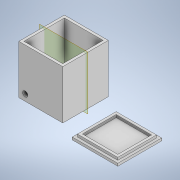
# Autodesk Inventor part: waterBallonHolder
Saved by Autodesk Inventor 2020 (Build 240168000, 168)
## iProperties
Created: 2022-09-13
Part Number: waterBallonHolder
Material: Generic
Document SubType Name: Modeling
Designer: iss
Density: 1 g/cm^3
Appearance: Default
Author: iss
Autodesk Inventor part; units mm, degrees
ref_plane "YZ Plane" through (0, 0, 0) normal (1, 0, 0) x (0, 1, 0)
ref_plane "XZ Plane" through (0, 0, 0) normal (0, 1, 0) x (-1, 0, 0)
ref_plane "XY Plane" through (0, 0, 0) normal (0, 0, 1) x (1, 0, 0)
sketch "Sketch1" plane through (0, 0, 0) normal (0, 1, 0) x (-1, 0, 0)
  line L0 (0, 0) -> (34.29, 0)
  line L1 (0, 0) -> (0, -35.56)
  line L2 (0, 0) -> (34.29, 0)
  line L3 (34.29, 0) -> (34.29, -35.56)
  line L4 (34.29, -35.56) -> (0, -35.56)
  line L5 (0, -35.56) -> (0, 0)
  dimension "d0" = 34.29
  dimension "d1" = 35.56
  constraints: 12 end point, 2 horizontal, 2 parallel, 1 perpendicular, 1 vertical
  measures "d0" distance of L0.start L0.end
  measures "d1" distance of L0.start L1.end
extrude "Extrusion1" add sketch "Sketch1" along normal blind 38.1
sketch "Sketch2" plane through (0, 38.1, 0) normal (0, 1, 0) x (1, 0, 0)
  line L0 (-34.29, 35.56) -> (-34.29, 0) projected
  line L1 (-34.29, 0) -> (0, 0) projected
  line L2 (0, 0) -> (0, 35.56) projected
  line L3 (0, 35.56) -> (-34.29, 35.56) projected
  line L4 (-32.29, 33.56) -> (-32.29, 2)
  line L5 (-32.29, 2) -> (-2, 2)
  line L6 (-2, 2) -> (-2, 33.56)
  line L7 (-2, 33.56) -> (-32.29, 33.56)
  dimension "d4" = 2
  constraints: 8 end point, 3 other
  measures "d4" distance between parallel lines of L3 L7
extrude "Extrusion2" cut sketch "Sketch2" against normal blind 36.1 contours L7 L6 L5 L4
sketch "Sketch3" plane through (0, 0, -35.56) normal (0, 0, -1) x (-1, 0, 0)
  line L0 (0, 0) -> (34.29, 0) projected
  line L1 (34.29, 0) -> (34.29, 38.1) projected
  line L2 (0, 38.1) -> (34.29, 38.1) projected
  line L3 (0, 0) -> (0, 38.1) projected
  line L4 (34.29, 0) -> (34.29, 38.1) projected
  line L5 (34.29, 0) -> (29.29, 0)
  line L6 (0, 0) -> (34.29, 0) projected
  line L7 (29.29, 0) -> (29.29, 5.0607)
  line L8 (2, 38.1) -> (32.29, 38.1) projected
  line L9 (2, 38.1) -> (2, 2) projected
  line L10 (2, 2) -> (32.29, 2) projected
  line L11 (32.29, 38.1) -> (32.29, 2) projected
  line L12 (32.29, 38.1) -> (32.29, 2) projected
  dimension "d7" = 5
  dimension "d8" = 5.0607
  constraints: 4 end point, 1 coincident, 1 point on line, 1 vertical
  measures "d7" distance of L0.end L5.end
  measures "d8" distance of L5.end L7.end
hole "Hole1" at (-29.29, 5.0607, -35.56) direction (0, 0, 1) diameter 4 depth 2
ref_plane "Work Plane1" through (-2, 38.1, -17.78) normal (0, 0, -1) x (-1, 0, 0)
mirror "Mirror1" about plane through (-2, 38.1, -17.78) normal (0, 0, -1) of "Hole1"
sketch "Sketch4" plane through (0, 0, 0) normal (0, 1, 0) x (-1, 0, 0)
  line L0 (32.29, -33.56) -> (2, -33.56) projected
  line L1 (2, -33.56) -> (2, -2) projected
  line L2 (2, -2) -> (32.29, -2) projected
  line L3 (32.29, -2) -> (32.29, -33.56) projected
  line L4 (34.29, -35.56) -> (34.29, 0) projected
  line L5 (34.29, 0) -> (0, 0) projected
  line L6 (0, 0) -> (0, -35.56) projected
  line L7 (0, -35.56) -> (34.29, -35.56) projected
  line L8 (-15.1723, 7.7342) -> (-50.7323, 7.7342)
  line L9 (-50.7323, 7.7342) -> (-50.7323, -26.5558)
  line L10 (-50.7323, -26.5558) -> (-15.1723, -26.5558)
  line L11 (-15.1723, -26.5558) -> (-15.1723, 7.7342)
  dimension "d17" = 35.56
  dimension "d18" = 34.29
  constraints: 8 end point, 2 parallel, 1 horizontal, 1 perpendicular
  measures "d17" distance of L9.end L10.end
  measures "d18" distance of L8.end L9.end
extrude "Extrusion3" add sketch "Sketch4" along normal blind 2 contours L11 L10 L9 L8
sketch "Sketch5" plane through (0, 2, 0) normal (0, 1, 0) x (1, 0, 0)
  line L0 (50.7323, -7.7342) -> (50.7323, 26.5558) projected
  line L1 (50.7323, 26.5558) -> (15.1723, 26.5558) projected
  line L2 (15.1723, 26.5558) -> (15.1723, -7.7342) projected
  line L3 (15.1723, -7.7342) -> (50.7323, -7.7342) projected
  line L4 (17.1723, 24.5558) -> (48.7323, 24.5558)
  line L5 (48.7323, 24.5558) -> (48.7323, -5.7342)
  line L6 (48.7323, -5.7342) -> (17.1723, -5.7342)
  line L7 (17.1723, -5.7342) -> (17.1723, 24.5558)
  line L8 (46.7323, 22.5558) -> (19.1723, 22.5558)
  line L9 (19.1723, 22.5558) -> (19.1723, -3.7342)
  line L10 (19.1723, -3.7342) -> (46.7323, -3.7342)
  line L11 (46.7323, -3.7342) -> (46.7323, 22.5558)
  point P0 (0, 0)
  dimension "d21" = 2
  dimension "d22" = 2
  constraints: 16 end point, 6 other
  measures "d21" distance between parallel lines of L1 L4
  measures "d22" distance between parallel lines of L4 L8
extrude "Extrusion4" add sketch "Sketch5" along normal blind 2 contours L4 L5 L6 L7
body "Solid1"
